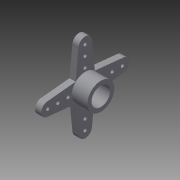
# Autodesk Inventor part: Ruderhorn_klein_Kreuz
Saved by Autodesk Inventor 2015 (Build 190159000, 159)
## iProperties
Created: 2015-02-12
Part Number: Ruderhorn_klein_Kreuz
Material: Generisch
Document SubType Name: Modeling
Designer: Raffael
Density: 1 g/cm^3
Appearance: Vorgabe
Author: Raffael
Autodesk Inventor part; units mm, degrees
ref_plane "YZ Plane" through (0, 0, 0) normal (1, 0, 0) x (0, 1, 0)
ref_plane "XZ Plane" through (0, 0, 0) normal (0, 1, 0) x (-1, 0, 0)
ref_plane "XY Plane" through (0, 0, 0) normal (0, 0, 1) x (1, 0, 0)
sketch "Skizze1" plane through (0, 0, 0) normal (1, 0, 0) x (0, 1, 0)
  circle A0 centre (0, 0) radius 4
  circle A1 centre (0, 0) radius 2.75
  arc A2 (-11, 2) -> (-11, -2) centre (-11, 0) ccw
  arc A3 (-2, -11) -> (2, -11) centre (0, -11) ccw
  arc A4 (11, -2) -> (11, 2) centre (11, 0) ccw
  arc A5 (2, 11) -> (-2, 11) centre (0, 11) ccw
  line L0 (0, 18.2) -> (0, -18.2) projected
  line L1 (-18.2, 0) -> (18.2, 0) projected
  line L2 (-18.2, 0) -> (18.2, 0) projected
  line L3 (0, -18.2) -> (0, 18.2) projected
  line L4 (2, 11) -> (2.8284, 2.8284)
  line L5 (-2, 11) -> (-2.8284, 2.8284)
  line L6 (-11, 2) -> (-2.8284, 2.8284)
  line L7 (-11, -2) -> (-2.8284, -2.8284)
  line L8 (-2, -11) -> (-2.8284, -2.8284)
  line L9 (2, -11) -> (2.8284, -2.8284)
  line L10 (2.8284, -2.8284) -> (11, -2)
  line L11 (11, 2) -> (2.8284, 2.8284)
  dimension "d0" = 8
  dimension "d1" = 5.5
  constraints: 16 end point, 12 point on circle, 6 centre point, 3 perpendicular, 2 coincident
  measures "d0" diameter of A0
  measures "d1" diameter of A1
extrude "Extrusion1" add sketch "Skizze1" along normal blind 1.8 contours L1 A4 L10 A0 | A0 L11 A4 L1 | A0 L0 A5 L4 | L9 A3 L0 A0 | A0 L5 A5 L0 | L0 A3 L8 A0 | A0 L1 A2 L6 | L7 A2 L1 A0
sketch "Skizze2" plane through (1.8, 0, 0) normal (1, 0, 0) x (0, 0, -1)
  circle A0 centre (0, 0) radius 2.75
  circle A1 centre (0, 0) radius 3.965
  dimension "d18" = 5.5
  constraints: 2 centre point, 2 coincident
  measures "d18" diameter of A0
extrude "Extrusion2" add sketch "Skizze2" along normal blind 4.6
sketch "Skizze3" plane through (1.8, 0, 0) normal (1, 0, 0) x (0, 0, -1)
  circle A0 centre (0, -11) radius 0.5
  circle A1 centre (0, -8) radius 0.5
  circle A2 centre (0, -5) radius 0.5
  circle A3 centre (0, 5) radius 0.5
  circle A4 centre (0, 8) radius 0.5
  circle A5 centre (0, 11) radius 0.5
  circle A6 centre (5, 0) radius 0.5
  circle A7 centre (8, 0) radius 0.5
  circle A8 centre (11, 0) radius 0.5
  circle A9 centre (-5, 0) radius 0.5
  circle A10 centre (-8, 0) radius 0.5
  circle A11 centre (-11, 0) radius 0.5
  point P0 (0, 0)
  dimension "d33" = 1
  dimension "d34" = 1
  dimension "d35" = 1
  dimension "d36" = 1
  dimension "d37" = 1
  dimension "d38" = 1
  dimension "d39" = 1
  dimension "d40" = 1
  dimension "d41" = 1
  dimension "d42" = 1
  dimension "d43" = 1
  dimension "d44" = 1
  constraints: 12 centre point, 4 coincident
  measures "d33" diameter of A0
  measures "d34" diameter of A1
  measures "d35" diameter of A2
  measures "d36" diameter of A3
  measures "d37" diameter of A4
  measures "d38" diameter of A5
  measures "d39" diameter of A6
  measures "d40" diameter of A7
  measures "d41" diameter of A8
  measures "d42" diameter of A9
  measures "d43" diameter of A10
  measures "d44" diameter of A11
extrude "Extrusion3" cut sketch "Skizze3" against normal blind 10
